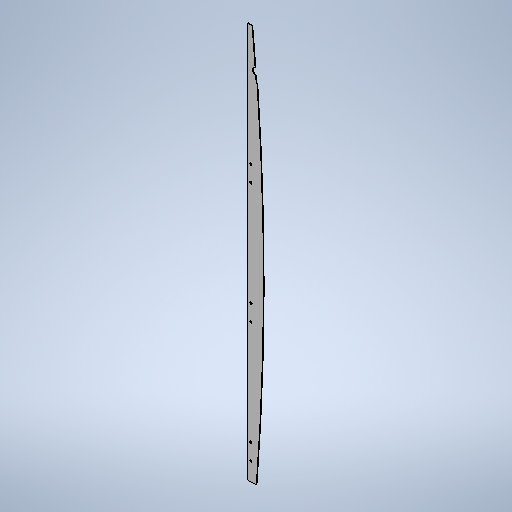
# Autodesk Inventor part: MSC 814 wall inner rib
Saved by Autodesk Inventor 2025.1 (Build 291241020, 241B)
## iProperties
Created: 2024-04-18
Part Number: MSC 814 wall inner rib
Material: AISI304
Document SubType Name: Sheet Metal
Designer: admin
Stock Number: МОО 813 стойка боковая жабры
Mass: 2919.69 g
Surface Area: 2571.84 cm^2
Volume: 364.962 cm^3
Density: 8 g/cm^3
Flat Pattern Width: 7.79022 cm
Flat Pattern Length: 197 cm
Flat Pattern Area: 1534.67 cm^2
Sheet Metal Rule: AISI304 3mm
Sheet Metal Width: 77.902 mm
Sheet Metal Length: 1970.000 mm
Sheet Metal Area: 153467.325 mm^2
Appearance: Default
Author: admin
Autodesk Inventor part; units mm, degrees
ref_plane "YZ Plane" through (0, 0, 0) normal (1, 0, 0) x (0, 1, 0)
ref_plane "XZ Plane" through (0, 0, 0) normal (0, 1, 0) x (-1, 0, 0)
ref_plane "XY Plane" through (0, 0, 0) normal (0, 0, 1) x (1, 0, 0)
sketch "Sketch1" plane through (0, 0, 0) normal (0, 0, 1) x (1, 0, 0)
  line L0 (0, 100) -> (0, 50) construction
  line L1 (0, 47) -> (0, 0) construction
  line L2 (0, 50) -> (0, 47) construction
  arc A0 (42, -1970) -> (25, 0) centre (-10972.0978, -1079.9722) ccw
  line L3 (42, -1970) -> (0, -1970)
  line L4 (0, -1970) -> (0, 0)
  line L5 (0, 0) -> (25, 0)
  line L6 (21, 0) -> (41.9305, -240)
  line L7 (41.9305, -240) -> (45.9305, -240)
  dimension "d115" = 3
  dimension "d131" = 11050
  dimension "d132" = 25
  dimension "d133" = 42
  dimension "d134" = 1970
  dimension "d145" = 4
  dimension "d146" = 240
  dimension "d147" = 4
  measures "d115" distance of L0.end L1.start
  measures "d131" radius of A0
  measures "d132" distance of L1.end L5.end
  measures "d133" distance of L3.start L3.end
  measures "d134" distance of L1.end L3.end
  measures "d145" distance of L6.end L7.end
  measures "d146" distance from line of L5 L6.end
  measures "d147" distance of L5.end L6.start
extrude "Plate3" add sketch "Sketch1" along normal blind 3 contours L3 L4 L5 L6 L7 A0
sketch "Sketch3" plane through (0, 0, 0) normal (0, 0, -1) x (-1, 0, 0)
  line L0 (0, 0) -> (0, -1970) construction
  line L1 (-21, 0) -> (0, 0) construction
  arc A0 (-45.9305, -240) -> (-42, -1970) centre (10972.0978, -1079.9722) ccw construction
  line L2 (0, -1970) -> (-42, -1970) projected
  circle A1 centre (-15, -600) radius 5.5
  line L3 (-41.9305, -240) -> (-21, 0) projected
  line L4 (-45.9305, -240) -> (-41.9305, -240) projected
  circle A2 centre (-15, -680) radius 5.5
  circle A3 centre (-37.5699, -190) radius 15
  circle A4 centre (-15, -1800) radius 5.5
  circle A5 centre (-15, -1880) radius 5.5
  circle A6 centre (-15, -1200) radius 5.5
  circle A7 centre (-15, -1280) radius 5.5
  dimension "d135" = 11
  dimension "d136" = 15
  dimension "d148" = 600
  dimension "d149" = 80
  dimension "d150" = 30
  dimension "d151" = 190
  dimension "d153" = 80
  dimension "d154" = 1200
  dimension "d157" = 80
  dimension "d159" = 1200
  constraints: 7 centre point, 6 vertical alignment, 4 equal radius, 1 point on line
  measures "d135" diameter of A1
  measures "d136" distance from line of L0 A1.centre
  measures "d148" distance from line of L1 A1.centre
  measures "d149" distance of A2.centre A1.centre
  measures "d150" diameter of A3
  measures "d151" distance from line of A3.centre L1
  measures "d153" distance of A5.centre A4.centre
  measures "d154" distance of A4.centre A1.centre
  measures "d157" distance of A7.centre A6.centre
  measures "d159" vertical distance of point (0, 0) A6.centre
extrude "Cut1" cut sketch "Sketch3" against normal blind 3
equation "\"BendReliefWidth\" = Thickness"
equation "\"BendReliefDepth\" = 0.5 * Thickness"
equation "\"CornerReliefSize\" = 4 * Thickness"
equation "\"MinimumRemnant\" = 2 * Thickness"
equation "\"GapSize\" = Thickness"
equation "\"Thickness\" = 3"
body "Solid4"
